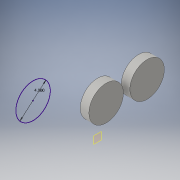
# Autodesk Inventor part: MarbleTemplate
Saved by Autodesk Inventor 2016 (Build 200138000, 138)
## iProperties
Created: 2017-01-25
Part Number: MarbleTemplate
Material: Generic
Document SubType Name: Modeling
Designer: Delta
Density: 1 g/cm^3
Appearance: Default
Author: Delta
Autodesk Inventor part; units mm, degrees
ref_plane "YZ Plane" through (0, 0, 0) normal (1, 0, 0) x (0, 1, 0)
ref_plane "XZ Plane" through (0, 0, 0) normal (0, 1, 0) x (-1, 0, 0)
ref_plane "XY Plane" through (0, 0, 0) normal (0, 0, 1) x (1, 0, 0)
sketch "Sketch7" plane through (0, 0, 0) normal (1, 0, 0) x (0, 1, 0)
  circle A0 centre (0, 0) radius 50.8
  dimension "d15" = 101.6
  constraints: 1 centre point, 1 coincident
  measures "d15" diameter of A0
ref_plane "Work Plane1" through (190.5, 0, 0) normal (1, 0, 0) x (0, 0, -1)
sketch "Sketch8" plane through (190.5, 0, 0) normal (1, 0, 0) x (0, 0, -1)
  line L0 (0, 0) -> (0, 101.6)
  circle A0 centre (0, 101.6) radius 50.8
  line L1 (0, 101.6) -> (120.65, 101.6)
  circle A1 centre (120.65, 101.6) radius 50.8
  point P0 (69.85, 101.6)
  point P1 (69.85, 101.6)
  dimension "d21" = 101.6
  dimension "d18" = 101.6
  dimension "d19" = 101.6
  dimension "d20" = 120.65
  constraints: 4 coincident, 4 end point, 1 centre point, 1 horizontal, 1 horizontal alignment, 1 point on line, 1 vertical, 2 other
  measures "d18" distance of L0.start L0.end
  measures "d19" diameter of A0
  measures "d20" distance of L1.start L1.end
extrude "Extrusion3" add sketch "Sketch8" along normal blind 25.4
body "Solid3"
